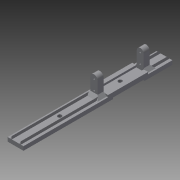
# Autodesk Inventor part: Top piece
Saved by Autodesk Inventor 2015 (Build 190159000, 159)
## iProperties
Created: 2014-11-22
Part Number: Top piece
Material: Generic
Document SubType Name: Modeling
Designer: jesse
Density: 1 g/cm^3
Appearance: Default
Author: jesse
Autodesk Inventor part; units mm, degrees
ref_plane "YZ Plane" through (0, 0, 0) normal (1, 0, 0) x (0, 1, 0)
ref_plane "XZ Plane" through (0, 0, 0) normal (0, 1, 0) x (-1, 0, 0)
ref_plane "XY Plane" through (0, 0, 0) normal (0, 0, 1) x (1, 0, 0)
sketch "Sketch1" plane through (0, 0, 0) normal (0, 0, 1) x (1, 0, 0)
  line L0 (10.119166, 6.643846) -> (35.519166, 6.643846)
  line L1 (35.519166, 6.643846) -> (35.519166, 0.293846)
  line L2 (35.519166, 0.293846) -> (10.119166, 0.293846)
  line L3 (10.119166, 0.293846) -> (10.119166, 6.643846)
  point P0 (0, 0)
  dimension "d0" = 25.4
  dimension "d1" = 6.35
  constraints: 8 end point, 2 parallel, 1 horizontal, 1 perpendicular
  measures "d0" distance of L1.end L2.end
  measures "d1" distance of L0.end L1.end
extrude "Extrusion1" add sketch "Sketch1" along normal blind 237.8075
sketch "Sketch2" plane through (10.119166, 6.643846, 0) normal (0, 1, 0) x (1, 0, 0)
  line L0 (0, 0) -> (25.4, 0)
  line L1 (0, 0) -> (0, -237.8075)
  line L2 (25.4, -237.8075) -> (0, -237.8075)
  line L3 (25.4, 0) -> (25.4, -237.8075)
  line L4 (12.7, 0) -> (12.7, -237.8075) construction
  line L5 (25.4, -237.8075) -> (0, -237.8075) construction
  line L6 (0, 0) -> (0, -237.8075) construction
  line L7 (0, -167.16375) -> (25.4, -167.16375) construction
  line L8 (0, -70.64375) -> (25.4, -70.64375) construction
  line L9 (25.4, 0) -> (25.4, -237.8075) construction
  circle A0 centre (12.7, -70.64375) radius 3.175
  circle A1 centre (12.7, -167.16375) radius 3.175
  line L10 (32.172126, -167.16375) -> (32.172126, -237.8075) construction
  line L11 (29.603984, -70.64375) -> (29.603984, 0) construction
  point P0 (-10.119166, 0)
  dimension "d6" = 6.35
  dimension "d7" = 6.35
  dimension "d10" = 96.52
  constraints: 10 end point, 8 point on line, 4 midpoint, 2 centre point, 2 parallel, 2 perpendicular, 1 vertical
  measures "d6" diameter of A0
  measures "d7" diameter of A1
  measures "d10" distance between parallel lines of L7 L8
extrude "Extrusion2" cut sketch "Sketch2" against normal through all contours A0 | A1
sketch "Sketch3" plane through (10.119166, 0.293846, 0) normal (-1, 0, 0) x (0, 0, 1)
  line L0 (44.84206, -2.796421) -> (94.995705, -2.796421)
  line L1 (94.995705, -2.796421) -> (94.995705, 2.208729)
  line L2 (94.995705, 2.208729) -> (44.84206, 2.208729)
  line L3 (44.84206, 2.208729) -> (44.84206, -2.796421)
  point P0 (0, -0.293846)
  constraints: 8 end point, 2 parallel, 1 horizontal, 1 perpendicular
extrude "Extrusion3" cut sketch "Sketch3" against normal through all
sketch "Sketch4" plane through (10.119166, 6.643846, 0) normal (0, 1, 0) x (1, 0, 0)
  line L0 (18.35, -38.735) -> (6.35, -38.735)
  line L1 (6.35, -102.735) -> (18.35, -102.735)
  line L2 (18.35, -38.735) -> (7.104998, -38.735)
  line L3 (7.104998, -38.735) -> (7.104998, -29.21)
  line L4 (7.104998, -29.21) -> (18.35, -29.21)
  line L5 (18.35, -29.21) -> (18.35, -38.735)
  line L6 (18.35, -102.735) -> (6.35, -102.735)
  line L7 (6.35, -102.735) -> (6.35, -112.26)
  line L8 (6.35, -112.26) -> (18.35, -112.26)
  line L9 (18.35, -112.26) -> (18.35, -102.735)
  point P0 (-10.119166, 0)
  dimension "d13" = 9.525
  dimension "d14" = 9.525
  constraints: 16 end point, 4 parallel, 2 horizontal, 2 perpendicular
  measures "d13" distance of L2.end L3.end
  measures "d14" distance of L7.end L6.end
extrude "Extrusion4" add sketch "Sketch4" along normal blind 30.1625
chamfer "Chamfer1" distance 4.7625 angle 45 2 edges at (22.8467, 6.6438, 29.21) (22.4692, 6.6438, 112.26)
sketch "Sketch5" plane through (16.469166, 36.806346, 112.26) normal (0, 0, 1) x (1, 0, 0)
  circle A0 centre (6, -22.1625) radius 1.35255
  circle A1 centre (6, -6.1625) radius 1.35255
  point P0 (-16.469166, -36.806346)
extrude "Extrusion5" cut sketch "Sketch5" against normal through all
fillet "Fillet1" radius 6.35 4 edges at (16.4692, 36.8063, 107.4975) (28.4692, 36.8063, 107.4975) (17.2242, 36.8063, 33.9725) (28.4692, 36.8063, 33.9725)
chamfer "Chamfer2" distance 4.7625 angle 45 4 edges at (16.4692, 6.6438, 109.8788) (28.4692, 6.6438, 109.8788) (28.4692, 6.6438, 31.5913) (17.2242, 6.6438, 31.5913)
sketch "Sketch6" plane through (10.119166, 6.643846, 0) normal (0, 1, 0) x (1, 0, 0)
  line L0 (25.4, -237.8075) -> (0, -237.8075)
  line L1 (18.692748, -237.8075) -> (21.155522, -237.8075)
  line L2 (21.155522, -225.1075) -> (21.155522, -112.051842)
  line L3 (21.155522, -112.051842) -> (18.692748, -112.051842)
  line L4 (18.692748, -112.051842) -> (18.692748, -225.1075)
  line L5 (6.707252, -237.8075) -> (4.244478, -237.8075)
  line L6 (4.244478, -225.1075) -> (4.244478, -112.051842)
  line L7 (4.244478, -112.051842) -> (6.707252, -112.051842)
  line L8 (6.707252, -112.051842) -> (6.707252, -225.1075)
  line L9 (25.4, 0) -> (25.4, -237.8075)
  line L10 (0, 0) -> (0, -237.8075)
  line L11 (21.155522, -171.841497) -> (25.4, -171.841497)
  line L12 (4.244478, -171.841497) -> (0, -171.841497)
  line L13 (20.86651, -0.289012) -> (18.403737, -0.289012)
  line L14 (18.403737, -12.7) -> (18.403737, -34.261512)
  line L15 (18.403737, -34.261512) -> (20.86651, -34.261512)
  line L16 (20.86651, -34.261512) -> (20.86651, -12.7)
  line L17 (7.104998, -29.21) -> (2.342498, -24.4475)
  line L18 (3.955467, -0.289012) -> (6.41824, -0.289012)
  line L19 (6.41824, -12.7) -> (6.41824, -28.523242)
  line L20 (6.41824, -28.523242) -> (3.955467, -28.523242)
  line L21 (3.955467, -28.523242) -> (3.955467, -12.7)
  line L22 (-2.54, -225.1075) -> (27.94, -225.1075)
  line L23 (27.94, -12.7) -> (-2.54, -12.7)
  point P0 (-10.119166, 0)
  constraints: 36 end point, 17 point on line, 8 parallel, 5 horizontal, 5 perpendicular, 2 collinear
sketch "Sketch6 outline for Extrusion6" plane through (10.119166, 6.643846, 0) normal (0, 1, 0) x (1, 0, 0)
  line L0 (6.41824, -28.523242) -> (6.41824, -12.7)
  line L1 (3.955467, -28.523242) -> (6.41824, -28.523242)
  line L2 (3.955467, -12.7) -> (3.955467, -28.523242)
  line L3 (6.41824, -12.7) -> (3.955467, -12.7)
  line L4 (18.403737, -12.7) -> (18.403737, -34.261512)
  line L5 (20.86651, -12.7) -> (18.403737, -12.7)
  line L6 (20.86651, -34.261512) -> (20.86651, -12.7)
  line L7 (18.403737, -34.261512) -> (20.86651, -34.261512)
  line L8 (21.155522, -225.1075) -> (21.155522, -112.051842)
  line L9 (21.155522, -112.051842) -> (18.692748, -112.051842)
  line L10 (18.692748, -112.051842) -> (18.692748, -225.1075)
  line L11 (18.692748, -225.1075) -> (21.155522, -225.1075)
  line L12 (6.707252, -112.051842) -> (4.244478, -112.051842)
  line L13 (4.244478, -112.051842) -> (4.244478, -225.1075)
  line L14 (4.244478, -225.1075) -> (6.707252, -225.1075)
  line L15 (6.707252, -225.1075) -> (6.707252, -112.051842)
extrude "Extrusion6" add sketch "Sketch6 outline for Extrusion6" along normal blind 4.7625 draft -20
sketch "Sketch7" plane through (10.119166, 6.643846, 0) normal (0, 1, 0) x (1, 0, 0)
  line L0 (18.35, -90.587941) -> (18.35, -50.882059) construction
  line L1 (6.35, -50.882059) -> (6.35, -90.587941) construction
  line L2 (18.35, -99.735) -> (18.35, -41.735) construction
  line L3 (6.35, -99.735) -> (18.35, -99.735) construction
  line L4 (6.35, -41.735) -> (6.35, -99.735) construction
  line L5 (18.35, -41.735) -> (6.35, -41.735) construction
  circle A0 centre (12.35, -54.735) radius 1.35255 construction
  circle A1 centre (12.35, -62.735) radius 1.35255 construction
  circle A2 centre (12.35, -78.735) radius 1.35255 construction
  circle A3 centre (12.35, -86.735) radius 1.35255 construction
  line L6 (1.5875, -102.735) -> (23.1125, -102.735)
  line L7 (23.1125, -38.735) -> (2.342498, -38.735)
  line L8 (25.4, 0) -> (25.4, -44.84206)
  line L9 (18.35, -102.735) -> (25.4, -102.735)
  line L10 (25.4, -102.735) -> (25.4, -38.735)
  line L11 (25.4, -38.735) -> (18.35, -38.735)
  line L12 (18.35, -38.735) -> (18.35, -102.735)
  line L13 (0, 0) -> (0, -237.8075)
  line L14 (0, -102.735) -> (6.35, -102.735)
  line L15 (6.35, -102.735) -> (6.35, -38.735)
  line L16 (6.35, -38.735) -> (0, -38.735)
  line L17 (0, -38.735) -> (0, -102.735)
  point P0 (-10.119166, 0)
  constraints: 16 end point, 5 point on line, 4 parallel, 2 horizontal, 2 perpendicular
extrude "Extrusion7" add sketch "Sketch7" along normal blind 3.175 contours L14 L13 L16 L7 L15 L6 | L12 L7 L11 L8 L10 L9 L6
sketch "Sketch8" plane through (35.519166, 6.643846, 38.735) normal (0, 0, -1) x (-1, 0, 0)
  line L0 (5.4625, 3.175) -> (2.2875, 0)
  line L1 (0, 3.175) -> (5.4625, 3.175)
  line L2 (0, 0) -> (0, 3.175)
  line L3 (2.2875, 0) -> (0, 0)
  line L4 (23.057502, 0) -> (19.882502, 3.175)
  line L5 (25.4, 0) -> (23.057502, 0)
  line L6 (25.4, 0) -> (25.4, 3.175)
  line L7 (19.882502, 3.175) -> (25.4, 3.175)
  point P0 (35.519166, -6.643846)
extrude "Extrusion8" cut sketch "Sketch8" against normal through all
body "Solid1"
